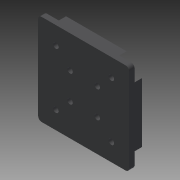
# Autodesk Inventor part: Bot 2.1
Saved by Autodesk Inventor 2015 (Build 190159000, 159)
## iProperties
Created: 2017-02-15
Part Number: Bot 2.1
Material: Generic
Document SubType Name: Modeling
Designer: Hampus
Density: 1 g/cm^3
Appearance: Gray
Author: Hampus
Autodesk Inventor part; units mm, degrees
note: some values were not read from the file. Chosen so that the rebuilt part matches the saved one: sketch regions of "Extrusion1".
ref_plane "YZ Plane" through (0, 0, 0) normal (1, 0, 0) x (0, 1, 0)
ref_plane "XZ Plane" through (0, 0, 0) normal (0, 1, 0) x (-1, 0, 0)
ref_plane "XY Plane" through (0, 0, 0) normal (0, 0, 1) x (1, 0, 0)
sketch "Grund" plane through (0, 0, 0) normal (0, 1, 0) x (-1, 0, 0)
  line L0 (-43, -43) -> (-7, -43)
  line L1 (-7, -43) -> (-7, -7)
  line L2 (-22.4779, -14.1174) -> (-8.3606, 0)
  line L3 (0, -8.61) -> (-13.9926, -22.6026)
  circle A0 centre (-32.4718, -17.6529) radius 1.5
  line L4 (-18.2353, -22.6026) -> (-22.4779, -18.36)
  line L5 (-22.4779, -14.1174) -> (-22.4779, -18.36)
  line L6 (-13.9926, -22.6026) -> (-18.2353, -22.6026)
  line L7 (-27.5221, -14.1174) -> (-27.5221, -18.36)
  line L8 (-31.7647, -22.6026) -> (-27.5221, -18.36)
  line L9 (-27.5221, -14.1174) -> (-41.6394, 0)
  line L10 (-36.0074, -22.6026) -> (-31.7647, -22.6026)
  line L11 (-50, -8.61) -> (-36.0074, -22.6026)
  line L12 (-27.5221, -35.8826) -> (-27.5221, -31.64)
  line L13 (-27.5221, -35.8826) -> (-41.6394, -50)
  line L14 (-36.0074, -27.3974) -> (-31.7647, -27.3974)
  line L15 (-31.7647, -27.3974) -> (-27.5221, -31.64)
  line L16 (-50, -41.39) -> (-36.0074, -27.3974)
  line L17 (-22.4779, -35.8826) -> (-22.4779, -31.64)
  line L18 (-22.4779, -35.8826) -> (-8.3606, -50)
  line L19 (-18.2353, -27.3974) -> (-22.4779, -31.64)
  line L20 (0, -41.39) -> (-13.9926, -27.3974)
  line L21 (-13.9926, -27.3974) -> (-18.2353, -27.3974)
  circle A1 centre (-32.4718, -32.3471) radius 1.5
  circle A2 centre (-40.25, -40.25) radius 1.5
  line L22 (-43, -7) -> (-43, -43)
  circle A3 centre (-17.5282, -17.6529) radius 1.5
  circle A4 centre (-17.5282, -32.3471) radius 1.5
  circle A5 centre (-9.75, -40.25) radius 1.5
  line L23 (-7, -7) -> (-43, -7)
  circle A6 centre (-9.75, -9.75) radius 1.5
  circle A7 centre (-40.25, -9.75) radius 1.5
  line L24 (0, 0) -> (0, -50)
  line L25 (0, -50) -> (-50, -50)
  line L26 (-50, -50) -> (-50, 0)
  line L27 (-50, 0) -> (0, 0)
  point P0 (-16.114, -25.276)
  point P1 (-24.5992, -33.7613)
  point P2 (-25.4008, -33.7613)
  point P3 (-33.886, -25.276)
  point P4 (-25.4008, -16.2387)
  point P5 (-33.886, -24.724)
  point P6 (-24.5992, -16.2387)
  point P7 (-16.114, -24.724)
  dimension "d0" = 36
  dimension "d1" = 36
  dimension "d4" = 3
  dimension "d5" = 3
  dimension "d6" = 3
  dimension "d7" = 3
  dimension "d9" = 50
  dimension "d10" = 50
  constraints: 56 end point, 12 point on line, 8 centre point, 2 parallel, 2 perpendicular, 1 horizontal
  measures "d0" distance of L0.start L0.end
  measures "d1" distance of L0.start L23.end
  measures "d4" diameter of A6
  measures "d5" diameter of A7
  measures "d6" diameter of A2
  measures "d7" diameter of A5
  measures "d9" distance of L24.start L24.end
  measures "d10" distance of L26.end L24.start
extrude "Extrusion1" add sketch "Grund" along normal blind 3
extrude "Extrusion2" add sketch "Grund" along normal blind 7 contours L13 L12 L15 L14 L16 L22 L11 L10 L8 L7 L9 L23 L2 L5 L4 L6 L3 L1 L20 L21 L19 L17 L18 L0 | L0 L18 L25 L13 | L16 L26 L11 L22 | L1 L3 L24 L20 | L9 L27 L2 L23
fillet "Fillet1" radius 2 4 edges at (50, 1.5, -50) (50, 1.5, 0) (0, 1.5, 0) (0, 1.5, -50)
body "Solid1"
